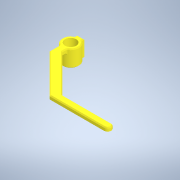
# Autodesk Inventor part: wing_lock
Saved by Autodesk Inventor 2021 (Build 250183000, 183)
## iProperties
Created: 2021-02-04
Part Number: wing_lock
Material: Generic
Document SubType Name: Modeling
Designer: Daniel
Density: 1 g/cm^3
Appearance: Default
Author: Daniel
Autodesk Inventor part; units mm, degrees
ref_plane "YZ Plane" through (0, 0, 0) normal (1, 0, 0) x (0, 1, 0)
ref_plane "XZ Plane" through (0, 0, 0) normal (0, 1, 0) x (-1, 0, 0)
ref_plane "XY Plane" through (0, 0, 0) normal (0, 0, 1) x (1, 0, 0)
sketch "Sketch1" plane through (0, 0, 0) normal (0, 1, 0) x (-1, 0, 0)
  arc A0 (-3.9997, -59.9493) -> (4, -60) centre (0, -60) ccw
  line L0 (0, 0) -> (-102, 0) construction
  line L1 (-3.9997, -4) -> (-102, -4)
  line L2 (-102, 4) -> (4, 4)
  arc A1 (-102, 4) -> (-102, -4) centre (-102, 0) ccw
  circle A2 centre (0, -60) radius 2.25
  line L3 (4, -60) -> (4, 4)
  circle A3 centre (0, -60) radius 6.375
  circle A4 centre (0, -60) radius 9.375
  line L4 (-85.873, 1) -> (-105.873, 1)
  line L5 (-105.873, -1) -> (-85.873, -1)
  line L6 (-85.873, -1) -> (-85.873, 1)
  line L7 (-3.9997, -59.9493) -> (-3.9997, -4)
  line L8 (-4, -68.4788) -> (4, -68.4788)
  line L9 (4, -68.4788) -> (4, -71.375)
  line L10 (4, -71.375) -> (-4, -71.375)
  line L11 (-4, -71.375) -> (-4, -68.4788)
  circle A5 centre (0, -60) radius 11.375 construction
  line L12 (-46.4261, -4) -> (-3.9997, -46.4264)
  line L13 (-43.1124, 4) -> (4, -43.1124)
  point P0 (-51, 0)
  point P1 (-8.5189, -5)
  point P2 (4, -51.5212)
  point P3 (-92.743, 0)
  point P4 (-3.9997, -51.521)
  point P5 (4, -55.0361)
  point P6 (-3.9997, -55.0358)
  point P7 (-3.9997, -35.1127)
  point P8 (-35.1124, -4)
  dimension "d9" = 4.5
  dimension "d24" = 4
  dimension "d29" = 12.75
  dimension "d30" = 3
  dimension "d46" = 102
  dimension "d48" = 2
  dimension "d49" = 20
  dimension "d50" = 1
  dimension "d52" = 60
  dimension "d53" = 7.9997
  dimension "d54" = 8
  dimension "d55" = 90
  dimension "d56" = 8
  dimension "d58" = 5
  dimension "d59" = 8
  dimension "d60" = 30
  dimension "d61" = 45
  constraints: 30 end point, 9 parallel, 8 point on circle, 6 centre point, 5 coincident, 5 point on line, 4 tangent, 2 perpendicular, 1 horizontal, 1 midpoint, 1 vertical alignment
  measures "d9" diameter of A2
  measures "d24" radius of A0
  measures "d29" diameter of A3
  measures "d30" radial gap between concentric circles of A4 A3
  measures "d46" distance of L0.start L0.end
  measures "d48" distance between parallel lines of L4 L5
  measures "d49" distance of L4.start L4.end
  measures "d50" distance between parallel lines of L0 L4
  measures "d52" distance of A0.centre point (0, 0)
  measures "d53" distance between parallel lines of L7 L3
  measures "d54" distance between parallel lines of L1 L2
  measures "d55" angle of L1 L7
  measures "d56" distance of L8.start L8.end
  measures "d58" radial gap between concentric circles of A3 A5
  measures "d59" distance between parallel lines of L13 L12
  measures "d60" distance from line of L1.start L12
  measures "d61" angle of L1 L12
extrude "Extrusion1" add sketch "Sketch1" along normal blind 4 contours L7 A4 L3 A3 | A3 L3 A4 L8 L7 | L7 L13 L3 A4 | L8 A4 | A4 L9 L10 L11 | L12 L1 L13 L7 | L1 A1 L5 L6 L4 L2 L13
sketch "Sketch7" plane through (0, 0, 0) normal (0, -1, 0) x (1, 0, 0)
  arc A0 (-4, -51.5212) -> (3.9997, -51.521) centre (0, -60) ccw projected
  circle A1 centre (0, -60) radius 6.4
  circle A2 centre (0, -60) radius 9.375
  line L0 (43.1124, 4) -> (102, 4) projected
  arc A3 (105.873, 1) -> (102, 4) centre (102, 0) ccw projected
  line L1 (102, -4) -> (46.4261, -4) projected
  arc A4 (4, -68.4788) -> (3.9997, -51.521) centre (0, -60) ccw projected
  line L2 (4, -68.4788) -> (4, -71.375) projected
  line L3 (4, -71.375) -> (-4, -71.375) projected
  line L4 (-4, -71.375) -> (-4, -68.4788) projected
  arc A5 (-4, -51.5212) -> (-4, -68.4788) centre (0, -60) ccw projected
  line L5 (46.4261, -4) -> (3.9997, -46.4264) projected
  line L6 (3.9997, -46.4264) -> (3.9997, -51.521) projected
  line L7 (-4, -51.5212) -> (-4, -43.1124) projected
  line L8 (-4, -43.1124) -> (43.1124, 4) projected
  line L9 (105.873, 1) -> (85.873, 1) projected
  line L10 (85.873, 1) -> (85.873, -1) projected
  line L11 (85.873, -1) -> (105.873, -1) projected
  arc A6 (102, -4) -> (105.873, -1) centre (102, 0) ccw projected
  point P0 (0, 0)
  point P1 (3.9997, -51.521)
  point P2 (-4, -68.4788)
  point P3 (4, -68.4788)
  point P4 (-4, -68.4788)
  point P5 (-4, -68.4788)
  point P6 (4, -68.4788)
  dimension "d31" = 12.8
  constraints: 2 centre point, 2 coincident, 1 concentric
  measures "d31" diameter of A1
extrude "Extrusion6" add sketch "Sketch7" along normal blind 15 contours A2 A0 | A0 L2 L3 L4
sketch "Sketch8" plane through (8.4512, 0, -71.375) normal (0, 0, 1) x (1, 0, 0)
  circle A0 centre (-8.4512, -7) radius 1.65
  line L0 (-17.8262, -15) -> (0.9238, -15) projected
  point P0 (-8.4512, 0)
  point P1 (-2.6893, 8)
  point P2 (-8.4512, -15)
  point P3 (-8.4512, -15)
  dimension "d34" = 3.3
  dimension "d47" = 8
  constraints: 2 vertical alignment, 1 centre point, 1 midpoint
  measures "d34" diameter of A0
  measures "d47" distance from line of L0 A0.centre
extrude "Extrusion7" cut sketch "Sketch8" along normal up to surface
fillet "Fillet2" radius 2 3 edges at (-0.0002, 0, -50.625) (-4, 2, -51.5212) (3.9997, 2, -51.521)
chamfer "Chamfer1" distance 1 angle 45 15 edges at (-9.3596, 4, -60.5379) (-4.2522, 4, -51.3083) (-4, 4, -46.7242) (9.3596, 4, -60.5378) (4.2519, 4, -51.3081) (3.9997, 4, -48.3812) (72.5562, 4, 4) (104.4495, 4, 3.1623) (104.4495, 4, -3.1623) (74.213, 4, -4) (4, 4, -69.9269) (-4, 4, -69.9269) (0, 4, -71.375) (25.2129, 4, -25.2132) (19.5562, 4, -19.5562)
chamfer "Chamfer2" distance 1 angle 45 5 edges at (-6.4, -15, -60) (0, -15, -50.625) (4, -15, -69.9269) (0, -15, -71.375) (-4, -15, -69.9269)
equation "\"d50\" = 0.5 * d48"
body "Solid1"
